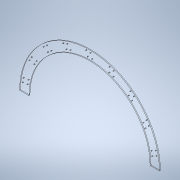
# Autodesk Inventor part: wheel2
Saved by Autodesk Inventor 2020.3 (Build 243373000, 373)
## iProperties
Created: 2020-11-01
Part Number: wheel2
Material: Generic
Document SubType Name: Modeling
Designer: Martijn
Density: 1 g/cm^3
Appearance: Default
Author: Martijn
Autodesk Inventor part; units mm, degrees
ref_plane "YZ Plane" through (0, 0, 0) normal (1, 0, 0) x (0, 1, 0)
ref_plane "XZ Plane" through (0, 0, 0) normal (0, 1, 0) x (-1, 0, 0)
ref_plane "XY Plane" through (0, 0, 0) normal (0, 0, 1) x (1, 0, 0)
sketch "Sketch1" plane through (0, 0, 0) normal (0, 0, 1) x (1, 0, 0)
  circle A0 centre (0, 0) radius 260
  circle A1 centre (0, 0) radius 300
  dimension "d0" = 600
  dimension "d1" = 40
  constraints: 2 centre point, 2 coincident
  measures "d0" diameter of A1
  measures "d1" radial gap between concentric circles of A1 A0
extrude "Extrusion1" add sketch "Sketch1" along normal blind 4
sketch "Sketch2" plane through (0, 0, 4) normal (0, 0, 1) x (1, 0, 0)
  line L0 (-300, 0) -> (300, 0)
  line L1 (300, 0) -> (300, -300)
  line L2 (300, -300) -> (-300, -300)
  line L3 (-300, -300) -> (-300, 0)
  circle A0 centre (0, 0) radius 300 projected
  line L4 (-420, 0) -> (420, 0) projected
  constraints: 8 end point, 3 tangent, 2 parallel, 1 collinear, 1 horizontal, 1 perpendicular
extrude "Extrusion2" cut sketch "Sketch2" against normal blind 10 contours L0 A0 picked at (-23.3445, -97.237)
sketch "Sketch3" plane through (0, 0, 4) normal (0, 0, 1) x (1, 0, 0)
  circle A0 centre (-288.2644, 34.2678) radius 1.5
  arc A1 (300, 0) -> (-300, 0) centre (0, 0) ccw projected
  circle A2 centre (-267.3724, 37.5767) radius 1.5
  line L0 (-420, 0) -> (420, 0) projected
  circle A3 centre (-284.9918, 52.8272) radius 1.5
  circle A4 centre (-264.0999, 56.1362) radius 1.5
  line L1 (-267.3724, 37.5767) -> (-288.2644, 34.2678)
  line L2 (-288.2644, 34.2678) -> (-284.9918, 52.8272)
  line L3 (-284.9918, 52.8272) -> (-264.0999, 56.1362)
  line L4 (-264.0999, 56.1362) -> (-267.3724, 37.5767)
  line L5 (-264.0999, 56.1362) -> (0, 0)
  line L6 (0, 0) -> (-267.3724, 37.5767)
  dimension "d6" = 3
  dimension "d7" = 3
  dimension "d9" = 270
  dimension "d11" = 3
  dimension "d12" = 3
  dimension "d14" = 270
  dimension "d21" = 109
  dimension "d22" = 20
  dimension "d23" = 8
  dimension "d24" = 12
  constraints: 12 end point, 4 centre point, 2 parallel
  measures "d6" diameter of A2
  measures "d7" diameter of A0
  measures "d9" distance of point (0, 0) L1.start
  measures "d11" diameter of A3
  measures "d12" diameter of A4
  measures "d14" distance of point (0, 0) L3.end
  measures "d21" angle of L1 L4
  measures "d22" distance between parallel lines of L2 L4
  measures "d23" angle of L0 L6
  measures "d24" angle of L0 L5
extrude "Extrusion3" cut sketch "Sketch3" against normal through all contours A0 L2 L1 | L1 L2 A0 | L1 L6 A2 | A2 L4 L1 | L2 L3 A3 | A3 L3 L2 | A2 L6 L4 | L4 L5 A4 | A4 L3 L4 | A4 L5 L3
pattern_circular "Circular Pattern1" count 9 over 160 about axis through (0, 0, 0) along (0, 0, -1) of "Extrusion3"
body "Solid1"
